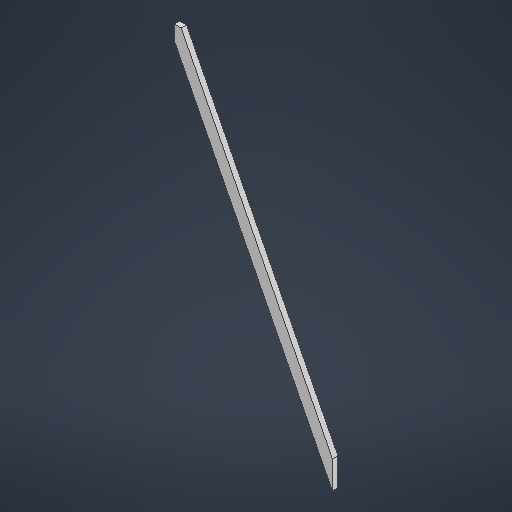
# Autodesk Inventor part: S_2x4x100.488
Saved by Autodesk Inventor 2026 (Build 300175000, 175)
## iProperties
Created: 2025-09-04
Part Number: S_2x4x100.488
Material: Generic
Document SubType Name: Modeling
Designer: trott
Density: 1 g/cm^3
Appearance: Default
Author: trott
Autodesk Inventor part; units mm, degrees
ref_plane "YZ Plane" through (0, 0, 0) normal (1, 0, 0) x (0, 1, 0)
ref_plane "XZ Plane" through (0, 0, 0) normal (0, 1, 0) x (-1, 0, 0)
ref_plane "XY Plane" through (0, 0, 0) normal (0, 0, 1) x (1, 0, 0)
sketch "Sketch1" plane through (0, 0, 0) normal (0, 0, 1) x (1, 0, 0)
  line L0 (-558.8, -2197.1) -> (558.8, -2197.1)
  line L1 (558.8, -2197.1) -> (558.8, 2197.1)
  line L2 (558.8, 2197.1) -> (-558.8, 2197.1)
  line L3 (-558.8, 2197.1) -> (-558.8, -2197.1)
  line L4 (-558.8, -2197.1) -> (558.8, 2197.1) construction
  line L5 (558.8, -2197.1) -> (-558.8, 2197.1) construction
  line L6 (-558.8, 0) -> (558.8, 0)
  line L7 (558.8, 0) -> (-558.8, -2197.1)
  line L8 (-519.1811, -2217.253) -> (-598.4189, -2176.947)
  line L9 (598.4189, -20.153) -> (519.1811, 20.153)
  line L10 (519.1811, 20.153) -> (-598.4189, -2176.947)
  line L11 (-519.1811, -2217.253) -> (598.4189, -20.153)
  line L12 (519.1811, 20.153) -> (558.8, 98.0402)
  line L13 (-558.8, 2197.1) -> (558.8, -2197.1) construction
  line L14 (558.8, 0) -> (-558.8, 2197.1)
  line L15 (-519.1811, 2217.253) -> (-598.4189, 2176.947)
  line L16 (598.4189, 20.153) -> (519.1811, -20.153)
  line L17 (519.1811, -20.153) -> (-598.4189, 2176.947)
  line L18 (-519.1811, 2217.253) -> (598.4189, 20.153)
  line L19 (519.1811, -20.153) -> (558.8, -98.0402)
  point P0 (0, 0)
  point P1 (558.8, 98.0402)
  point P2 (-508.9298, 2197.1)
  point P3 (-558.8, 2099.0598)
  point P4 (558.8, -98.0402)
  point P5 (558.8, -98.0402)
  point P6 (508.9298, 0)
  point P7 (-558.8, -2099.0598)
  point P8 (-508.9298, -2197.1)
  dimension "d0" = 1117.6
  dimension "d1" = 4394.2
  dimension "d3" = 88.9
  dimension "d4" = 88.9
  constraints: 40 end point, 6 midpoint, 5 symmetric about line, 3 perpendicular, 3 point on line, 2 parallel, 1 horizontal
  measures "d0" distance of L2.end L1.end
  measures "d1" distance of L0.end L1.end
  measures "d3" distance of L8.start L8.end
  measures "d4" distance of L9.start L9.end
extrude "Extrusion1" add sketch "Sketch1" along normal blind 38.1 contours L19 L16 L7 | L7 L1 L19 | L10 L9 L6 | L17 L3 L14 L12 L10 | L6 L16 L17 | L14 L12 L1 | L9 L12 L14 | L12 L14 L2 L18
body "Solid1"
